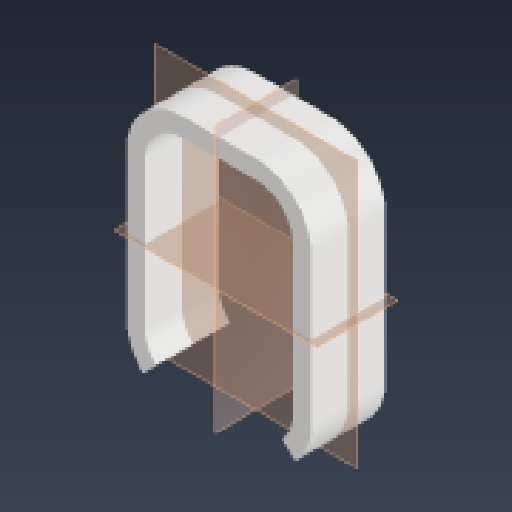
# Autodesk Inventor part: Козырёк_для_камеры
Saved by Autodesk Inventor 2023.2 (Build 272271030, 271C)
## iProperties
Created: 2025-10-07
Part Number: Козырёк_для_камеры
Material: Типовые
Document SubType Name: Modeling
Designer: Олег Коноваленко
Density: 1 g/cm^3
Appearance: По умолчанию
Author: Олег Коноваленко
Autodesk Inventor part; units mm, degrees
sketch "Эскиз2" plane through (0, 0, 0) normal (0, 0, 1) x (1, 0, 0)
  arc A0 (20, 20) -> (10, 30) centre (10, 20) ccw projected
  line L0 (20, -20) -> (20, 20) projected
  arc A1 (10, -30) -> (20, -20) centre (10, -20) ccw projected
  line L1 (-10, -30) -> (10, -30) projected
  arc A2 (-20, -20) -> (-10, -30) centre (-10, -20) ccw projected
  line L2 (-20, 20) -> (-20, -20) projected
  arc A3 (-10, 30) -> (-20, 20) centre (-10, 20) ccw projected
  line L3 (10, 30) -> (-10, 30) projected
  arc A4 (-10, 35) -> (-25, 20) centre (-10, 20) ccw
  line L4 (-25, 20) -> (-25, -20)
  arc A5 (-25, -20) -> (-10, -35) centre (-10, -20) ccw
  line L5 (-10, -35) -> (10, -35)
  arc A6 (10, -35) -> (25, -20) centre (10, -20) ccw
  line L6 (25, -20) -> (25, 20)
  arc A7 (25, 20) -> (10, 35) centre (10, 20) ccw
  line L7 (10, 35) -> (-10, 35)
  line L8 (17.0711, -27.0711) -> (20.6066, -30.6066)
  line L9 (0, 53.3492) -> (0, -53.3492) construction
  line L10 (-17.0711, -27.0711) -> (-20.6066, -30.6066)
  dimension "d8" = 5
  constraints: 12 end point, 11 point on circle, 4 centre point, 2 symmetric about line, 7 other
  measures "d8" distance between parallel lines of L3 L7
extrude "Выдавливание2" add sketch "Эскиз2" along normal mid plane 50 contours A0 L3 A3 L2 A2 L10 A5 L4 A4 L7 A7 L6 A6 L8 A1 L0
